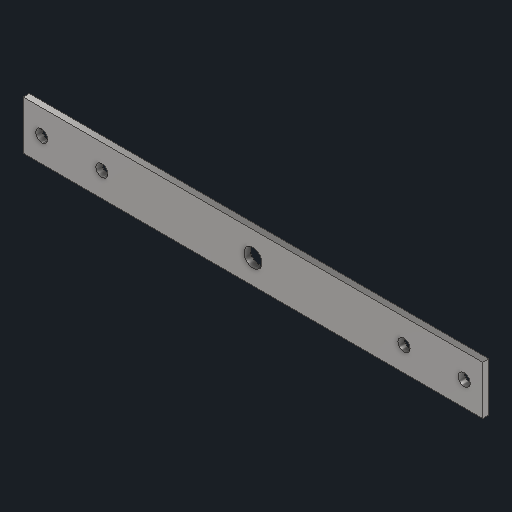
# Autodesk Inventor part: ThrustArmWash
Saved by Autodesk Inventor 2024 (Build 280153000, 153)
## iProperties
Created: 2025-02-08
Part Number: ThrustArmWash
Material: Stainless Steel
Document SubType Name: Modeling
Designer: Tommy Rohmann
Density: 8 g/cm^3
Appearance: Semi-Polished
Author: Tommy Rohmann
Autodesk Inventor part; units mm, degrees
ref_plane "YZ Plane" through (0, 0, 0) normal (1, 0, 0) x (0, 1, 0)
ref_plane "XZ Plane" through (0, 0, 0) normal (0, 1, 0) x (-1, 0, 0)
ref_plane "XY Plane" through (0, 0, 0) normal (0, 0, 1) x (1, 0, 0)
sketch "ACMEThrustNut" plane through (0, 0, 0) normal (0, 0, 1) x (1, 0, 0)
  line L0 (-68.4054, 438.7087) -> (-68.4054, 413.3087)
  line L1 (-62.0554, 438.7087) -> (-43.0054, 438.7087)
  line L2 (-43.0054, 438.7087) -> (-43.0054, 413.3087)
  line L3 (-43.0054, 413.3087) -> (-62.0554, 413.3087)
  line L4 (-74.7554, 438.7087) -> (-93.8054, 438.7087)
  line L5 (-93.8054, 438.7087) -> (-93.8054, 413.3087)
  line L6 (-93.8054, 413.3087) -> (-74.7554, 413.3087)
  line L7 (-74.7554, 413.3087) -> (-74.7554, 438.7087)
  line L8 (-74.7554, 438.7087) -> (-62.0554, 438.7087)
  line L9 (-62.0554, 438.7087) -> (-62.0554, 413.3087)
  line L10 (-62.0554, 413.3087) -> (-74.7554, 413.3087)
  line L11 (-93.8054, 426.0087) -> (-43.0054, 426.0087)
  arc A0 (-53.8911, 429.1837) -> (-53.8911, 422.8337) centre (-53.8911, 426.0087) ccw
  arc A1 (-51.4721, 422.8337) -> (-51.4721, 429.1837) centre (-51.4721, 426.0087) ccw
  line L12 (-51.4721, 429.1837) -> (-53.8911, 429.1837)
  line L13 (-51.4721, 422.8337) -> (-53.8911, 422.8337)
  arc A2 (-82.9197, 422.8337) -> (-82.9197, 429.1837) centre (-82.9197, 426.0087) ccw
  line L14 (-85.3387, 422.8337) -> (-82.9197, 422.8337)
  arc A3 (-85.3387, 429.1837) -> (-85.3387, 422.8337) centre (-85.3387, 426.0087) ccw
  line L15 (-85.3387, 429.1837) -> (-82.9197, 429.1837)
  dimension "d427" = 25.4
  dimension "d428" = 12.7
  dimension "d429" = 19.05
  dimension "d437" = 6.35
  dimension "d438" = 10.8857
  dimension "d439" = 6.35
  dimension "d440" = 8.4667
  measures "d427" distance of L7.start L7.end
  measures "d428" distance of L7.end L8.end
  measures "d429" distance of L8.end L1.end
  measures "d437" diameter of A0
  measures "d438" distance from line of L2 A0.centre
  measures "d439" diameter of A1
  measures "d440" distance from line of L2 A1.centre
sketch "ThrustArmWash" plane through (0, 0, 0) normal (0, 0, 1) x (1, 0, 0)
  line L0 (-122.2582, 479.0809) -> (-96.8582, 479.0809)
  line L1 (-96.8582, 479.0809) -> (-96.8582, 453.6809)
  line L2 (-96.8582, 453.6809) -> (-122.2582, 453.6809)
  line L3 (-216.8732, 453.6809) -> (-122.2582, 453.6809)
  line L4 (-122.2582, 453.6809) -> (-122.2582, 479.0809)
  line L5 (-122.2582, 479.0809) -> (-216.8732, 479.0809)
  circle A0 centre (-216.8732, 466.3809) radius 4.7625
  line L6 (-216.8732, 453.6809) -> (-216.8732, 479.0809)
  circle A1 centre (-137.982, 466.3809) radius 3.175
  circle A2 centre (-106.5344, 466.3809) radius 3.175
  line L7 (-122.2582, 479.0809) -> (-122.2582, 453.6809)
  line L8 (-115.9082, 479.0809) -> (-96.8582, 479.0809)
  line L9 (-96.8582, 479.0809) -> (-96.8582, 453.6809)
  line L10 (-96.8582, 453.6809) -> (-115.9082, 453.6809)
  line L11 (-128.6082, 479.0809) -> (-147.6582, 479.0809)
  line L12 (-147.6582, 479.0809) -> (-147.6582, 453.6809)
  line L13 (-147.6582, 453.6809) -> (-128.6082, 453.6809)
  line L14 (-128.6082, 453.6809) -> (-128.6082, 479.0809)
  line L15 (-128.6082, 479.0809) -> (-115.9082, 479.0809)
  line L16 (-115.9082, 479.0809) -> (-115.9082, 453.6809)
  line L17 (-115.9082, 453.6809) -> (-128.6082, 453.6809)
  line L18 (-147.6582, 466.3809) -> (-96.8582, 466.3809)
  arc A3 (-107.7439, 469.5559) -> (-107.7439, 463.2059) centre (-107.7439, 466.3809) ccw
  arc A4 (-105.3249, 463.2059) -> (-105.3249, 469.5559) centre (-105.3249, 466.3809) ccw
  line L19 (-105.3249, 469.5559) -> (-107.7439, 469.5559)
  line L20 (-105.3249, 463.2059) -> (-107.7439, 463.2059)
  arc A5 (-136.7725, 463.2059) -> (-136.7725, 469.5559) centre (-136.7725, 466.3809) ccw
  line L21 (-139.1916, 463.2059) -> (-136.7725, 463.2059)
  arc A6 (-139.1916, 469.5559) -> (-139.1916, 463.2059) centre (-139.1916, 466.3809) ccw
  line L22 (-139.1916, 469.5559) -> (-136.7725, 469.5559)
  dimension "d425" = 94.615
  dimension "d426" = 25.4
  dimension "d430" = 9.525
  measures "d425" distance of L3.start L3.end
  measures "d426" distance of L3.end L4.end
  measures "d430" diameter of A0
derived "LAYOUT.ipt"
sketch "Sketch1" plane through (0, 0, 0) normal (0, 0, 1) x (1, 0, 0)
  line L0 (-122.2582, 479.0809) -> (-96.8582, 479.0809)
  line L1 (-96.8582, 479.0809) -> (-96.8582, 453.6809)
  line L2 (-96.8582, 453.6809) -> (-122.2582, 453.6809)
  line L3 (-216.8732, 453.6809) -> (-122.2582, 453.6809)
  line L4 (-122.2582, 453.6809) -> (-122.2582, 479.0809)
  line L5 (-122.2582, 479.0809) -> (-216.8732, 479.0809)
  circle A0 centre (-216.8732, 466.3809) radius 4.7625
  line L6 (-216.8732, 453.6809) -> (-216.8732, 479.0809)
  circle A1 centre (-137.982, 466.3809) radius 3.175
  circle A2 centre (-106.5344, 466.3809) radius 3.175
  line L7 (-122.2582, 479.0809) -> (-122.2582, 453.6809)
  line L8 (-115.9082, 479.0809) -> (-96.8582, 479.0809)
  line L9 (-96.8582, 479.0809) -> (-96.8582, 453.6809)
  line L10 (-96.8582, 453.6809) -> (-115.9082, 453.6809)
  line L11 (-128.6082, 479.0809) -> (-147.6582, 479.0809)
  line L12 (-147.6582, 479.0809) -> (-147.6582, 453.6809)
  line L13 (-147.6582, 453.6809) -> (-128.6082, 453.6809)
  line L14 (-128.6082, 453.6809) -> (-128.6082, 479.0809)
  line L15 (-128.6082, 479.0809) -> (-115.9082, 479.0809)
  line L16 (-115.9082, 479.0809) -> (-115.9082, 453.6809)
  line L17 (-115.9082, 453.6809) -> (-128.6082, 453.6809)
  line L18 (-147.6582, 466.3809) -> (-96.8582, 466.3809)
  arc A3 (-107.7439, 469.5559) -> (-107.7439, 463.2059) centre (-107.7439, 466.3809) ccw
  arc A4 (-105.3249, 463.2059) -> (-105.3249, 469.5559) centre (-105.3249, 466.3809) ccw
  line L19 (-105.3249, 469.5559) -> (-107.7439, 469.5559)
  line L20 (-105.3249, 463.2059) -> (-107.7439, 463.2059)
  arc A5 (-136.7725, 463.2059) -> (-136.7725, 469.5559) centre (-136.7725, 466.3809) ccw
  line L21 (-139.1916, 463.2059) -> (-136.7725, 463.2059)
  arc A6 (-139.1916, 469.5559) -> (-139.1916, 463.2059) centre (-139.1916, 466.3809) ccw
  line L22 (-139.1916, 469.5559) -> (-136.7725, 469.5559)
  point P0 (-216.8732, 471.1434)
  point P1 (-216.8732, 461.6184)
extrude "Extrusion1" add sketch "Sketch1" along normal blind 3.175 contours L0 L16 L18 L4 | L4 L18 L14 L5 | L0 L1 L18 A4 L19 A3 L16 | L18 L16 L2 L4 | L4 L3 L14 L18 | L14 L18 A5 L22 A6 L12 L5 | L18 A3 L20 A4 L1 L2 L16 | L14 L3 L12 L18 A6 L21 A5 | L12 L3 L6 A0 L5 | A3 L19 A2 L18 | L18 A2 L20 A3 | A5 L21 A1 L18 | L18 A1 L22 A5 | A4 L20 A2 L18 | L18 A2 L19 A4 | A6 L22 A1 L18 | L18 A1 L21 A6
mirror "Mirror1" about plane through (-216.8732, 479.0809, 0) normal (-1, 0, 0)
body "Solid1"
